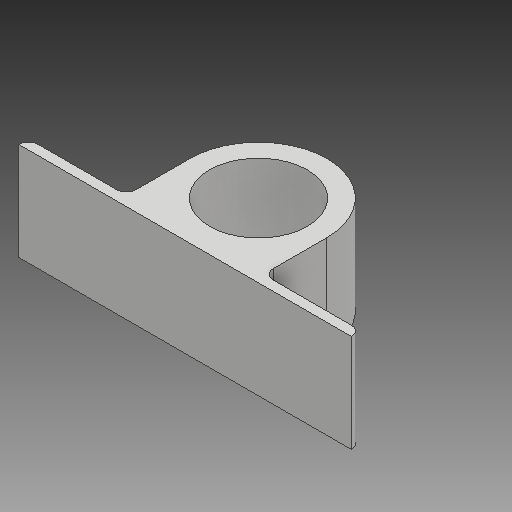
# Autodesk Inventor part: asKogellager
Saved by Autodesk Inventor 2017 (Build 210142000, 142)
## iProperties
Created: 2017-02-17
Part Number: asKogellager
Material: Generic
Document SubType Name: Modeling
Designer: Koen
Density: 1 g/cm^3
Appearance: Default
Author: Koen
Autodesk Inventor part; units mm, degrees
ref_plane "YZ Plane" through (0, 0, 0) normal (1, 0, 0) x (0, 1, 0)
ref_plane "XZ Plane" through (0, 0, 0) normal (0, 1, 0) x (-1, 0, 0)
ref_plane "XY Plane" through (0, 0, 0) normal (0, 0, 1) x (1, 0, 0)
sketch "Sketch1" plane through (0, 0, 0) normal (0, 0, 1) x (1, 0, 0)
  line L0 (-190, -896.7461) -> (-190, -1116.7461) projected
  line L1 (-190, -1116.7461) -> (-710, -1116.7461) projected
  line L2 (-710, -1116.7461) -> (-710, -896.7461) projected
  line L3 (-710, -896.7461) -> (-190, -896.7461) projected
  line L4 (-150, -20) -> (150, -20) projected
  line L5 (150, -20) -> (150, 20) projected
  line L6 (150, 20) -> (-190, 20) projected
  line L7 (-190, 20) -> (-190, -856.7461) projected
  line L8 (-190, -856.7461) -> (-710, -856.7461) projected
  line L9 (-710, -856.7461) -> (-710, 20) projected
  arc A0 (-710, 20) -> (-1028.8395, 243.2539) centre (-947.5818, 20) ccw projected
  line L10 (-1028.8395, 243.2539) -> (-1015.1587, 205.6661) projected
  arc A1 (-750, 20) -> (-1015.1587, 205.6661) centre (-947.5818, 20) ccw projected
  line L11 (-750, 20) -> (-750, -1156.7461) projected
  line L12 (-750, -1156.7461) -> (-150, -1156.7461) projected
  line L13 (-150, -1156.7461) -> (-150, -20) projected
  line L14 (-634, -1116.7461) -> (-634, -1116.7461)
  line L15 (-632, -1114.7461) -> (-616, -1114.7461)
  line L16 (-614, -1112.7461) -> (-614, -1101.7461)
  arc A2 (-586, -1101.7461) -> (-614, -1101.7461) centre (-600, -1101.7461) ccw
  line L17 (-586, -1101.7461) -> (-586, -1112.7461)
  line L18 (-584, -1114.7461) -> (-568, -1114.7461)
  line L19 (-566, -1116.7461) -> (-566, -1116.7461)
  circle A3 centre (-600, -1101.7461) radius 10
  arc A4 (-586, -1112.7461) -> (-584, -1114.7461) centre (-584, -1112.7461) ccw
  arc A5 (-616, -1114.7461) -> (-614, -1112.7461) centre (-616, -1112.7461) ccw
  arc A6 (-566, -1116.7461) -> (-568, -1114.7461) centre (-568, -1116.7461) ccw
  arc A7 (-632, -1114.7461) -> (-634, -1116.7461) centre (-632, -1116.7461) ccw
  point P0 (0, 0)
  point P1 (-634, -1114.7461)
  point P2 (-614, -1114.7461)
  point P3 (-586, -1114.7461)
  point P4 (-566, -1114.7461)
  dimension "d0" = 20
  dimension "d1" = 2
  dimension "d2" = 4
  dimension "d3" = 20
  dimension "d4" = 20
  dimension "d5" = 15
  dimension "d6" = 150
  dimension "d7" = 2
  constraints: 12 end point, 12 point on line, 10 point on circle, 10 tangent, 6 centre point, 4 perpendicular, 3 equal radius, 1 coincident, 1 parallel
  measures "d0" diameter of A3
  measures "d1" distance of L14.start point (-634, -1114.746)
  measures "d2" radial gap between concentric circles of A3 A2
  measures "d3" distance of point (-634, -1114.746) point (-614, -1114.746)
  measures "d4" distance of point (-586, -1114.746) point (-566, -1114.746)
  measures "d5" distance from line of L1 A3.centre
  measures "d6" distance from line of L11 A2.centre
  measures "d7" radius of A4
extrude "Extrusion1" add sketch "Sketch1" against normal blind 20 contours L1 A7 L15 A5 L16 A2 L17 A4 L18 A6
equation "\"d4\" = d3"
body "Solid1"
